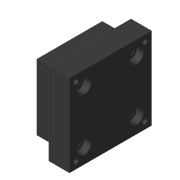
# Autodesk Inventor part: OCT_SpiegelAdapter_MovingSt.
Saved by Autodesk Inventor 2022 (Build 260153000, 153)
## iProperties
Created: 2023-06-26
Part Number: OCT_SpiegelAdapter_MovingSt.
Material: Generisch
Document SubType Name: Modeling
Designer: UC2
Density: 1 g/cm^3
Appearance: Vorgabe
Author: UC2
Autodesk Inventor part; units mm, degrees
ref_plane "YZ Plane" through (0, 0, 0) normal (1, 0, 0) x (0, 1, 0)
ref_plane "XZ Plane" through (0, 0, 0) normal (0, 1, 0) x (-1, 0, 0)
ref_plane "XY Plane" through (0, 0, 0) normal (0, 0, 1) x (1, 0, 0)
sketch "Skizze1" plane through (0, 0, 0) normal (1, 0, 0) x (0, 1, 0)
  line L0 (20, 20) -> (-20, 20)
  line L1 (-20, 20) -> (-20, -20)
  line L2 (-20, -20) -> (20, -20)
  line L3 (20, -20) -> (20, 20)
  line L4 (20, 20) -> (-20, -20) construction
  line L5 (-20, 20) -> (20, -20) construction
  point P0 (0, 0)
  dimension "d0" = 40
  dimension "d1" = 40
  constraints: 12 end point, 2 midpoint, 2 parallel, 1 horizontal, 1 perpendicular
  measures "d0" distance of L2.end L1.end
  measures "d1" distance of L1.end L0.end
extrude "Extrusion1" add sketch "Skizze1" along normal blind 25
sketch "Skizze2" plane through (25, 0, 0) normal (1, 0, 0) x (0, 0, -1)
  line L0 (-25, 25) -> (25, 25)
  line L1 (25, 25) -> (25, -25)
  line L2 (25, -25) -> (-25, -25)
  line L3 (-25, -25) -> (-25, 25)
  line L4 (-25, 25) -> (25, -25) construction
  line L5 (25, 25) -> (-25, -25) construction
  point P0 (0, 0)
  dimension "d4" = 50
  dimension "d5" = 50
  constraints: 12 end point, 2 midpoint, 2 parallel, 1 horizontal, 1 perpendicular
  measures "d4" distance of L1.end L2.end
  measures "d5" distance of L0.end L1.end
extrude "Extrusion2" add sketch "Skizze2" against normal blind 12.5
sketch "Skizze3" plane through (25, 0, 0) normal (1, 0, 0) x (0, 0, -1)
  point P0 (0, 0)
  point P1 (21, -21)
  point P2 (-21, -21)
  point P3 (-21, 21)
  point P4 (21, 21)
  point P5 (16, -16)
  point P6 (-16, -16)
  point P7 (-16, 16)
  point P8 (16, 16)
hole "Bohrung1" at (25, -21, -21) at (25, -21, 21) at (25, 21, 21) at (25, 21, -21) at (25, -16, -16) at (25, -16, 16) at (25, 16, 16) at (25, 16, -16) direction (-1, 0, 0) diameter 2.8 depth 230
sketch "Skizze4" plane through (25, 0, 0) normal (1, 0, 0) x (0, 0, -1)
  circle A0 centre (-16, 16) radius 1.4 projected
  circle A1 centre (16, -16) radius 1.4 projected
  circle A2 centre (-21, 21) radius 1.4 projected
  circle A3 centre (21, -21) radius 1.4 projected
  circle A4 centre (-21, -21) radius 1.4 projected
  circle A5 centre (21, 21) radius 1.4 projected
  circle A6 centre (-16, -16) radius 1.4 projected
  circle A7 centre (16, 16) radius 1.4 projected
  line L0 (-25, -25) -> (25, -25) projected
  line L1 (25, -25) -> (25, 25) projected
  line L2 (25, 25) -> (-25, 25) projected
  line L3 (-25, 25) -> (-25, -25) projected
  circle A8 centre (-16, 16) radius 1.4 projected
  circle A9 centre (16, 16) radius 1.4 projected
  circle A10 centre (16, -16) radius 1.4 projected
  point P0 (0, 0)
  constraints: 4 coincident
hole "Bohrung2" at (25, 16, 16) at (25, 16, -16) at (25, -16, -16) at (25, -16, 16) direction (-1, 0, 0) diameter 4.2 depth 230 counterbore diameter 8 counterbore depth 4
